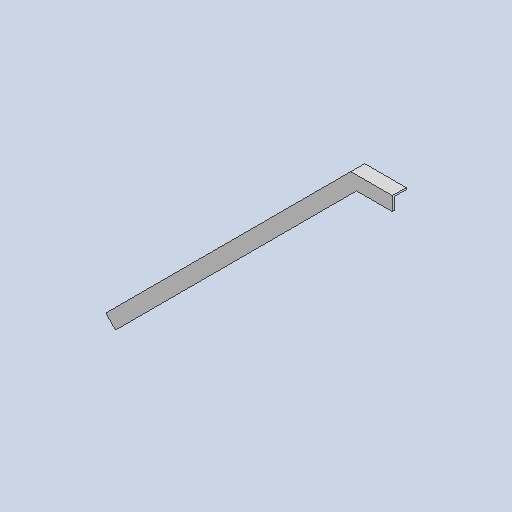
# Autodesk Inventor part: DiagR
Saved by Autodesk Inventor 2023 (Build 270158030, 158C)
## iProperties
Created: 2022-06-27
Part Number: DiagR
Material: Generic
Document SubType Name: Modeling
Designer: jeremyy
Density: 1 g/cm^3
Appearance: Default
Author: jeremyy
Autodesk Inventor part; units mm, degrees
ref_plane "YZ Plane" through (0, 0, 0) normal (1, 0, 0) x (0, 1, 0)
ref_plane "XZ Plane" through (0, 0, 0) normal (0, 1, 0) x (-1, 0, 0)
ref_plane "XY Plane" through (0, 0, 0) normal (0, 0, 1) x (1, 0, 0)
sketch "Sketch1" plane through (0, 0, 0) normal (0, 0, 1) x (1, 0, 0)
  line L0 (0, 0) -> (224.5064, 224.5064)
  line L1 (0, 0) -> (317.5, 0) construction
  line L2 (224.5064, 224.5064) -> (262.6064, 224.5064)
  line L3 (262.6064, 224.5064) -> (262.6064, 211.8064)
  line L4 (262.6064, 211.8064) -> (229.7669, 211.8064)
  line L5 (229.7669, 211.8064) -> (224.5064, 224.5064)
  line L6 (0, 0) -> (8.9803, -8.9803)
  line L7 (8.9803, -8.9803) -> (229.7669, 211.8064)
  line L8 (0, 0) -> (1.1225, -1.1225)
  line L9 (1.1225, -1.1225) -> (225.164, 222.9189)
  line L10 (262.6064, 224.5064) -> (262.6064, 222.9189)
  line L11 (262.6064, 222.9189) -> (225.164, 222.9189)
  dimension "d0" = 317.5
  dimension "d1" = 45
  dimension "d2" = 38.1
  dimension "d3" = 12.7
  dimension "d4" = 12.7
  dimension "d5" = 90
  dimension "d8" = 1.5875
  dimension "d9" = 1.5875
  constraints: 24 end point, 4 perpendicular, 3 point on line, 2 horizontal, 1 equal length
  measures "d0" distance of L0.start L0.end
  measures "d1" angle of L1 L0
  measures "d2" distance of L0.end L2.end
  measures "d3" distance of L2.end L3.end
  measures "d4" distance of L0.start L6.end
  measures "d5" angle of L7 L6
  measures "d8" distance of L0.start L8.end
  measures "d9" distance of L2.end L10.end
extrude "Extrusion1" add sketch "Sketch1" along normal blind 1.5875
extrude "Extrusion2" add sketch "Sketch1" against normal blind 11.1125 contours L0 L5 L9 L6 | L2 L3 L11 L5
body "Solid1"
